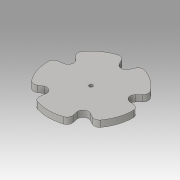
# Autodesk Inventor part: gear wheel
Saved by Autodesk Inventor 2016 (Build 200138000, 138)
## iProperties
Created: 2015-11-24
Part Number: gear wheel
Material: Generic
Document SubType Name: Modeling
Designer: Delta
Density: 1 g/cm^3
Appearance: Default
Author: Delta
Autodesk Inventor part; units mm, degrees
ref_plane "YZ Plane" through (0, 0, 0) normal (1, 0, 0) x (0, 1, 0)
ref_plane "XZ Plane" through (0, 0, 0) normal (0, 1, 0) x (-1, 0, 0)
ref_plane "XY Plane" through (0, 0, 0) normal (0, 0, 1) x (1, 0, 0)
sketch "Sketch1" plane through (0, 0, 0) normal (0, 1, 0) x (-1, 0, 0)
  circle A0 centre (0, 0) radius 76.2
  dimension "d0" = 152.4
  constraints: 2 coincident, 1 centre point
  measures "d0" diameter of A0
extrude "Extrusion1" add sketch "Sketch1" along normal blind 11.43
sketch "Sketch2" plane through (0, 11.43, 0) normal (0, 1, 0) x (1, 0, 0)
  circle A0 centre (0, 0) radius 76.2 projected
  line L0 (0.1023, 76.1999) -> (0.1023, 63.4999) construction
  arc A1 (-8.3552, 59.1187) -> (8.4222, 58.8626) centre (0.1023, 63.4999) ccw
  line L1 (8.4222, 58.8626) -> (15.4584, 74.6155)
  line L2 (-8.3552, 59.1187) -> (-16.2911, 74.4382)
  dimension "d3" = 12.7
  dimension "d4" = 19.05
  dimension "d16" = 31.75
  constraints: 6 end point, 5 point on circle, 1 centre point, 1 coincident, 1 equal length, 1 tangent, 1 vertical
  measures "d3" distance of L0.start L0.end
  measures "d4" diameter of A1
  measures "d16" distance of L2.end L1.end
extrude "Extrusion2" cut sketch "Sketch2" against normal through all contours L1 A1 L2 A0 picked at (1.6562, 64.6745)
fillet "Fillet1" radius 9.525 1 edges at (-16.2911, 5.715, -74.4382)
fillet "Fillet2" radius 9.525 1 edges at (15.4584, 5.715, -74.6155)
pattern_circular "Circular Pattern1" count 5 over 360 about axis through (0, -10, 0) along (0, 1, 0) of "Extrusion2", "Fillet1", "Fillet2"
sketch "Sketch4" plane through (0, 0, 0) normal (0, -1, 0) x (1, 0, 0)
  circle A0 centre (0, 0) radius 3.175
  dimension "d19" = 6.35
  constraints: 1 centre point, 1 coincident
  measures "d19" diameter of A0
hole "Hole1" at (0, 0, 0) direction (0, 1, 0) diameter 6.35 end through all
body "Solid1"
